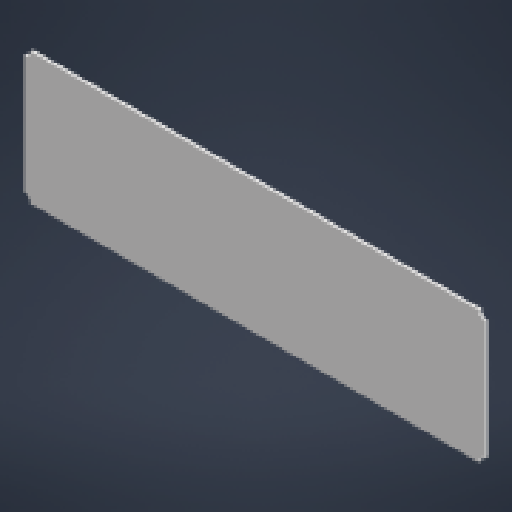
# Autodesk Inventor part: ypanel
Saved by Autodesk Inventor 2025.1 (Build 291241020, 241B)
## iProperties
Created: 2024-09-23
Part Number: ypanel
Material: Generic
Document SubType Name: Modeling
Designer: techn
Density: 1 g/cm^3
Appearance: Default
Author: techn
Autodesk Inventor part; units mm, degrees
ref_plane "YZ Plane" through (0, 0, 0) normal (1, 0, 0) x (0, 1, 0)
ref_plane "XZ Plane" through (0, 0, 0) normal (0, 1, 0) x (-1, 0, 0)
ref_plane "XY Plane" through (0, 0, 0) normal (0, 0, 1) x (1, 0, 0)
sketch "Sketch1" plane through (0, 0, 0) normal (0, 0, 1) x (1, 0, 0)
  line L0 (0, 0) -> (6, 0) projected
  line L1 (6, 0) -> (6, 120) projected
  line L2 (0, 120) -> (6, 120) projected
  line L3 (0, 0) -> (0, 120) projected
  line L4 (0, -6) -> (-440, -6) projected
  line L5 (0, -6) -> (0, 0) projected
  line L6 (-440, 0) -> (0, 0) projected
  line L7 (-440, -6) -> (-440, 0) projected
  line L8 (0, 126) -> (-440, 126) projected
  line L9 (-440, 126) -> (-440, 120) projected
  line L10 (-440, 120) -> (0, 120) projected
  line L11 (0, 120) -> (0, 126) projected
  line L12 (-446, 120) -> (-440, 120) projected
  line L13 (-440, 120) -> (-440, 0) projected
  line L14 (-446, 0) -> (-440, 0) projected
  line L15 (-446, 120) -> (-446, 0) projected
  line L16 (0, 120) -> (-440, 120)
  line L17 (-440, 120) -> (-440, 0)
  line L18 (-440, 0) -> (0, 0)
  line L19 (0, 0) -> (0, 120)
  line L20 (0, 118) -> (4, 118)
  line L21 (4, 118) -> (4, 2)
  line L22 (4, 2) -> (0, 2)
  line L23 (-438, 120) -> (-438, 124)
  line L24 (-438, 124) -> (-2, 124)
  line L25 (-2, 124) -> (-2, 120)
  line L26 (-438, 0) -> (-438, -4)
  line L27 (-438, -4) -> (-2, -4)
  line L28 (-2, -4) -> (-2, 0)
  line L29 (-440, 2) -> (-444, 2)
  line L30 (-444, 2) -> (-444, 118)
  line L31 (-444, 118) -> (-440, 118)
  point P0 (-456.0051, 134.3667)
  point P1 (-456.0051, 4.3667)
  point P2 (-6.0051, 134.3667)
  point P3 (-2, 0)
  dimension "d3" = 2
  dimension "d4" = 2
  dimension "d5" = 2
  dimension "d6" = 2
  constraints: 32 end point, 2 parallel, 1 horizontal, 1 perpendicular, 8 other
  measures "d3" distance between parallel lines of L1 L21
  measures "d4" distance between parallel lines of L8 L24
  measures "d5" distance between parallel lines of L4 L27
  measures "d6" distance between parallel lines of L15 L30
extrude "Extrusion1" add sketch "Sketch1" along normal blind 3 contours L6 L13 L10 L3 | L3 L20 L21 L22 | L28 L27 L26 L6 | L10 L23 L24 L25 | L29 L30 L31 L13
body "Solid1"
